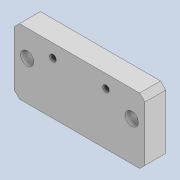
# Autodesk Inventor part: 0008-10-059
Saved by Autodesk Inventor 2020 (Build 240168000, 168)
## iProperties
Created: 2020-01-28
Part Number: 0008-10-059
Material: Generic
Document SubType Name: Modeling
Designer: iuliu
Density: 1 g/cm^3
Appearance: Default
Author: iuliu
Autodesk Inventor part; units mm, degrees
ref_plane "YZ Plane" through (0, 0, 0) normal (1, 0, 0) x (0, 1, 0)
ref_plane "XZ Plane" through (0, 0, 0) normal (0, 1, 0) x (-1, 0, 0)
ref_plane "XY Plane" through (0, 0, 0) normal (0, 0, 1) x (1, 0, 0)
sketch "Sketch1" plane through (0, 0, 0) normal (0, 0, 1) x (1, 0, 0)
  line L0 (0, 25) -> (50, 25)
  line L1 (50, 25) -> (50, 5)
  line L2 (35, 0) -> (0, 0)
  line L3 (0, 0) -> (0, 25)
  line L4 (35, 5) -> (50, 5)
  line L5 (35, 0) -> (35, 5)
  circle A0 centre (5, 15) radius 2.5
  circle A1 centre (45, 15) radius 2.5
  line L6 (25, 21.4836) -> (25, 16.0198) construction
  circle A2 centre (14.85, 20) radius 1.25
  circle A3 centre (35.15, 20) radius 1.25
  line L7 (35, 5) -> (50, 5)
  line L8 (50, 5) -> (50, 0)
  line L9 (50, 0) -> (35, 0)
  line L10 (35, 0) -> (35, 5)
  point P0 (25, 18.7517)
  point P1 (25, 25)
  dimension "d0" = 25
  dimension "d1" = 50
  dimension "d2" = 35
  dimension "d3" = 20
  dimension "d4" = 5
  dimension "d5" = 5
  dimension "d6" = 5
  dimension "d7" = 10
  dimension "d8" = 2.5
  dimension "d9" = 2.5
  dimension "d10" = 5
  dimension "d11" = 20.3
  constraints: 22 end point, 4 centre point, 4 collinear, 4 parallel, 3 horizontal, 2 horizontal alignment, 2 midpoint, 2 perpendicular, 1 coincident, 1 equal radius, 1 symmetric about line, 1 vertical, 1 vertical alignment
  measures "d0" distance of L2.end L0.start
  measures "d1" distance of L0.start L0.end
  measures "d2" distance between parallel lines of L3 L5
  measures "d3" distance between parallel lines of L4 L0
  measures "d4" diameter of A0
  measures "d5" distance from line of L3 A0.centre
  measures "d6" distance from line of L1 A1.centre
  measures "d7" distance from line of A1.centre L0
  measures "d8" diameter of A2
  measures "d9" diameter of A3
  measures "d10" distance from line of A3.centre L0
  measures "d11" distance of A3.centre A2.centre
extrude "Extrusion1" add sketch "Sketch1" along normal blind 8
chamfer "Chamfer1" distance 2 angle 45 4 edges at (0, 0, 4) (50, 25, 4) (0, 25, 4) (50, 0, 4)
body "Solid1"
